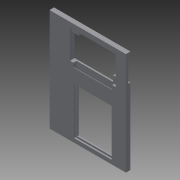
# Autodesk Inventor part: DisplayMid2
Saved by Autodesk Inventor 2014 SP1 (Build 180222100, 222)
## iProperties
Created: 2014-03-24
Part Number: DisplayMid2
Material: Generic
Document SubType Name: Modeling
Designer: patrigg
Density: 1 g/cm^3
Appearance: Default
Author: patrigg
Autodesk Inventor part; units mm, degrees
ref_plane "YZ Plane" through (0, 0, 0) normal (1, 0, 0) x (0, 1, 0)
ref_plane "XZ Plane" through (0, 0, 0) normal (0, 1, 0) x (-1, 0, 0)
ref_plane "XY Plane" through (0, 0, 0) normal (0, 0, 1) x (1, 0, 0)
sketch "Sketch2" plane through (0, 0, 0) normal (0, 1, 0) x (-1, 0, 0)
  line L0 (-33.5, -45) -> (33.5, -45)
  line L1 (33.5, -45) -> (33.5, 45)
  line L2 (33.5, 45) -> (-33.5, 45)
  line L3 (-33.5, 45) -> (-33.5, -45)
  line L4 (-33.5, -45) -> (33.5, 45) construction
  line L5 (33.5, -45) -> (-33.5, 45) construction
  point P0 (0, 0)
  dimension "d0" = 67
  dimension "d1" = 90
  constraints: 12 end point, 2 midpoint, 2 parallel, 1 horizontal, 1 perpendicular
  measures "d0" distance of L2.end L1.end
  measures "d1" distance of L1.end L0.end
extrude "Extrusion1" add sketch "Sketch2" along normal blind 4
sketch "Sketch3" plane through (0, 4, 0) normal (0, 1, 0) x (1, 0, 0)
  line L0 (33.5, 45) -> (-33.5, 45) projected
  line L1 (-14.5, -9.5) -> (23.5, -9.5)
  line L2 (23.5, -9.5) -> (23.5, 43)
  line L3 (23.5, 43) -> (-14.5, 43)
  line L4 (-14.5, 43) -> (-14.5, -9.5)
  line L5 (-14.5, -9.5) -> (23.5, 43) construction
  line L6 (23.5, -9.5) -> (-14.5, 43) construction
  line L7 (33.5, -45) -> (33.5, 45) projected
  point P0 (0, 0)
  point P1 (4.5, 16.75)
  dimension "d4" = 38
  dimension "d5" = 52.5
  dimension "d6" = 2
  dimension "d104" = 10
  constraints: 12 end point, 2 midpoint, 2 parallel, 1 horizontal, 1 perpendicular
  measures "d4" distance of L3.end L2.end
  measures "d5" distance of L2.end L1.end
  measures "d6" distance between parallel lines of L0 L3
  measures "d104" distance between parallel lines of L7 L2
extrude "Extrusion2" cut sketch "Sketch3" against normal blind 2.75
sketch "Sketch4" plane through (0, 1.25, 0) normal (0, 1, 0) x (1, 0, 0)
  line L0 (23.5, -9.5) -> (-14.5, -9.5) projected
  line L1 (23.5, 43) -> (23.5, -9.5) projected
  line L2 (-14.5, 43) -> (23.5, 43) projected
  line L3 (-14.5, -9.5) -> (-14.5, 43) projected
  line L4 (-12, 41.5) -> (21, 41.5)
  line L5 (21, 41.5) -> (21, 0.5)
  line L6 (21, 0.5) -> (-12, 0.5)
  line L7 (-12, 0.5) -> (-12, 41.5)
  line L8 (-12, 41.5) -> (21, 0.5) construction
  line L9 (21, 41.5) -> (-12, 0.5) construction
  point P0 (0, 0)
  point P1 (4.5, 21)
  dimension "d9" = 10
  dimension "d10" = 1.5
  dimension "d11" = 2.5
  dimension "d12" = 2.5
  constraints: 12 end point, 2 midpoint, 2 parallel, 1 horizontal, 1 perpendicular
  measures "d9" distance between parallel lines of L0 L6
  measures "d10" distance between parallel lines of L2 L4
  measures "d11" distance between parallel lines of L1 L5
  measures "d12" distance between parallel lines of L3 L7
extrude "Extrusion3" cut sketch "Sketch4" against normal blind 2.5 contours L4 L5 L6 L7
sketch "Sketch5" plane through (0, 4, 0) normal (0, 1, 0) x (1, 0, 0)
  line L0 (23.5, 43) -> (23.5, -9.5) projected
  line L1 (23.5, -9.5) -> (-14.5, -9.5) projected
  line L2 (-14.5, -9.5) -> (-14.5, 43) projected
  line L3 (-12.5, -15.5) -> (-12.5, -9.5)
  line L4 (21.5, -15.5) -> (21.5, -9.5)
  line L5 (33.5, 45) -> (-33.5, 45) projected
  line L6 (-12.5, -15.5) -> (21.5, -15.5)
  point P0 (0, 0)
  dimension "d18" = 2
  dimension "d19" = 2
  constraints: 6 end point, 2 perpendicular, 2 point on line, 1 parallel
  measures "d18" distance between parallel lines of L3 L2
  measures "d19" distance between parallel lines of L0 L4
extrude "Extrusion4" cut sketch "Sketch5" against normal blind 0.25
sketch "Sketch12" plane through (0, 4, 0) normal (0, 1, 0) x (1, 0, 0)
  line L0 (21.5, -15.5) -> (-12.5, -15.5) projected
  line L1 (-33.5, -45) -> (33.5, -45) projected
  line L2 (-15.5, -40.5) -> (24.5, -40.5)
  line L3 (24.5, -40.5) -> (24.5, -15.5)
  line L4 (24.5, -15.5) -> (-15.5, -15.5)
  line L5 (-15.5, -15.5) -> (-15.5, -40.5)
  line L6 (-15.5, -40.5) -> (24.5, -15.5) construction
  line L7 (24.5, -40.5) -> (-15.5, -15.5) construction
  line L8 (23.5, 43) -> (23.5, -9.5) projected
  point P0 (0, 0)
  point P1 (4.5, -28)
  point P2 (4.5, -28)
  point P3 (0, -45)
  dimension "d58" = 40
  dimension "d59" = 25
  dimension "d105" = 1
  constraints: 12 end point, 4 midpoint, 2 parallel, 1 collinear, 1 horizontal, 1 perpendicular
  measures "d58" distance of L4.end L3.end
  measures "d59" distance of L3.end L2.end
  measures "d105" distance between parallel lines of L8 L3
extrude "Extrusion10" cut sketch "Sketch12" against normal blind 4
sketch "Sketch13" plane through (24.5, 4, 15.5) normal (-1, 0, 0) x (0, 0, 1)
  line L0 (0, 0) -> (25, 0) projected
  line L1 (0, 0) -> (0, -4) projected
  line L2 (25, -4) -> (0, -4) projected
  line L3 (6, 0) -> (6, -4)
  line L4 (0, -2.2) -> (6, -2.2)
  point P0 (-15.5, -4)
  dimension "d67" = 6
  dimension "d74" = 1.8
  constraints: 4 end point, 4 point on line, 2 perpendicular
  measures "d67" distance between parallel lines of L3 L1
  measures "d74" distance between parallel lines of L2 L4
sketch "Sketch14" plane through (-15.5, 4, 40.5) normal (1, 0, 0) x (0, 0, -1)
  line L0 (0, 0) -> (25, 0) projected
  line L1 (0, 0) -> (0, -4)
  line L2 (4.0418, -2.2) -> (4.0418, 0)
  line L3 (25, -4) -> (0, -4) projected
  line L4 (0, -2.2) -> (4.0418, -2.2)
  point P0 (40.5, -4)
  point P1 (0, -2)
  dimension "d79" = 1.8
  constraints: 6 end point, 2 perpendicular, 2 point on line, 1 midpoint
  measures "d79" distance between parallel lines of L3 L4
extrude "Extrusion13" add sketch "Sketch13" along normal blind 4 contours L0 L3 L4 L1
extrude "Extrusion14" add sketch "Sketch14" along normal blind 6
sketch "Sketch16" plane through (0, 3.75, 0) normal (0, 1, 0) x (1, 0, 0)
  line L0 (-12.5, -15.5) -> (-12.5, -9.5) projected
  line L1 (20.5, -15.5) -> (-12.5, -15.5) projected
  line L2 (21.5, -15.5) -> (20.5, -15.5) projected
  line L3 (21.5, -9.5) -> (21.5, -15.5) projected
  line L4 (-12.5, -9.5) -> (21.5, -9.5) projected
  point P0 (0, 0)
extrude "Extrusion15" cut sketch "Sketch16" against normal up to next
sketch "Sketch17" plane through (21.5, 4, 9.5) normal (-1, 0, 0) x (0, 0, 1)
  line L0 (0, -2.75) -> (0, -4) projected
  line L1 (6, -4) -> (0, -4) projected
  line L2 (6, -2.2) -> (6, -4) projected
  line L3 (6, 0) -> (6, -2.2) projected
  line L4 (0, -2.75) -> (-1.7339, -2.75) construction
  line L5 (5, -4) -> (7.1842, -4) construction
  line L6 (0, -2.75) -> (5, -4) construction
  arc A0 (2.3486, -3.3) -> (0, -2.75) centre (0, -8.0397) ccw
  line L7 (0, -2.75) -> (0, 0) projected
  line L8 (2.3486, -4) -> (2.3486, -3.3)
  line L9 (0, 0) -> (6, 0) projected
  line L10 (0, -1.25) -> (6, -1.25)
  point P0 (-9.5, -4)
  dimension "d82" = 1
  dimension "d86" = 0.7
  dimension "d95" = 1.25
  constraints: 10 end point, 4 point on line, 2 parallel, 2 perpendicular, 2 point on circle, 1 centre point, 1 tangent
  measures "d82" distance from line of L2 L5.start
  measures "d86" distance of L8.start L8.end
  measures "d95" distance between parallel lines of L10 L9
extrude "Extrusion16" add sketch "Sketch17" along normal up to next contours A0 L8 L1 L0 | L7 L9 L3 L10
fillet "Fillet5" radius 1 1 edges at (4.5, 0.7, 11.8486)
sketch "Sketch18" plane through (23.5, 4, -43) normal (-1, 0, 0) x (0, 0, 1)
  line L0 (0, 0) -> (52.5, 0) projected
  line L1 (0, 0) -> (0, -2.75) projected
  line L2 (52.5, 0) -> (52.5, -2.75) projected
  line L3 (0, -1.25) -> (52.5, -1.25)
  line L4 (1.5, -2.75) -> (1.5, -4) projected
  line L5 (42.5, -2.75) -> (42.5, -4) projected
  dimension "d88" = 1.25
  constraints: 2 end point, 2 point on line, 1 perpendicular
  measures "d88" distance between parallel lines of L3 L0
extrude "Extrusion17" add sketch "Sketch18" along normal up to next
sketch "Sketch21" plane through (0, 4, 0) normal (0, 1, 0) x (1, 0, 0)
  line L0 (21, 41.5) -> (-12, 41.5) projected
  line L1 (21, 0.5) -> (21, 41.5) projected
  line L2 (-12, 41.5) -> (-12, 0.5) projected
  line L3 (-12, 0.5) -> (21, 0.5) projected
  point P0 (0, 0)
extrude "Extrusion19" cut sketch "Sketch21" against normal up to next
sketch "Sketch23" plane through (0, 4, 0) normal (0, 1, 0) x (1, 0, 0)
  line L0 (24.5, -21.5) -> (24.5, -40.5) projected
  line L1 (24.5, -40.5) -> (-9.5, -40.5) projected
  line L2 (33.5, -45) -> (33.5, 45) projected
  line L3 (24.5, -21.5) -> (33.5, -21.5)
  line L4 (24.5, -38.5) -> (33.5, -38.5)
  point P0 (0, 0)
  dimension "d106" = 2
  constraints: 4 end point, 3 point on line, 1 parallel, 1 perpendicular
  measures "d106" distance between parallel lines of L4 L1
extrude "Extrusion21" cut sketch "Sketch23" against normal blind 2
body "Solid1"
